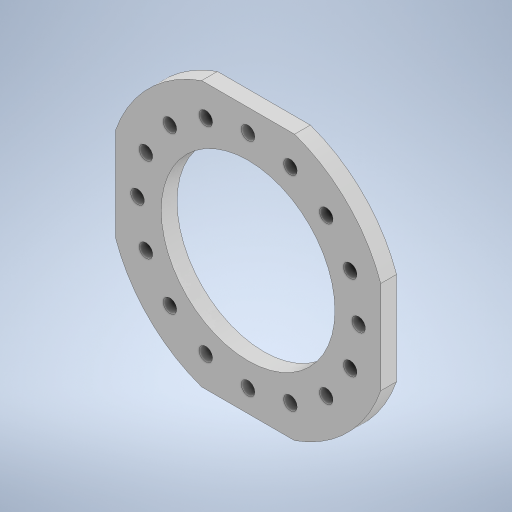
# Autodesk Inventor part: 감속기어1 - 하우징 커버
Saved by Autodesk Inventor 2023 (Build 270158000, 158)
## iProperties
Created: 2022-06-21
Part Number: 감속기어1 - 하우징 커버
Material: 일반
Document SubType Name: Modeling
Designer: user
Density: 1 g/cm^3
Appearance: 기본값
Author: user
Autodesk Inventor part; units mm, degrees
ref_plane "YZ Plane" through (0, 0, 0) normal (1, 0, 0) x (0, 1, 0)
ref_plane "XZ Plane" through (0, 0, 0) normal (0, 1, 0) x (-1, 0, 0)
ref_plane "XY Plane" through (0, 0, 0) normal (0, 0, 1) x (1, 0, 0)
sketch "스케치1" plane through (0, 0, 0) normal (0, 0, 1) x (1, 0, 0)
  circle A0 centre (0, 0) radius 44.5
  line L0 (-42, -42) -> (42, -42)
  line L1 (42, -42) -> (42, 42)
  line L2 (42, 42) -> (-42, 42)
  line L3 (-42, 42) -> (-42, -42)
  line L4 (-42, -42) -> (42, 42) construction
  line L5 (42, -42) -> (-42, 42) construction
  circle A1 centre (0, 0) radius 27.5
  point P0 (-42, 14.7054)
  point P1 (-42, -14.7054)
  point P2 (-14.7054, -42)
  point P3 (14.7054, -42)
  point P4 (42, -14.7054)
  point P5 (42, 14.7054)
  point P6 (14.7054, 42)
  point P7 (-14.7054, 42)
  dimension "d0" = 89
  dimension "d1" = 84
  dimension "d2" = 84
  dimension "d3" = 55
  constraints: 12 end point, 2 centre point, 2 coincident, 2 midpoint, 2 parallel, 1 horizontal, 1 perpendicular
  measures "d0" diameter of A0
  measures "d1" distance of L2.end L1.end
  measures "d2" distance of L1.end L0.end
  measures "d3" diameter of A1
extrude "돌출1" add sketch "스케치1" along normal blind 5 contours L1 A0 L0 L3 L2
sketch "스케치4" plane through (0, 0, 5) normal (0, 0, 1) x (1, 0, 0)
  circle A0 centre (0, 35) radius 2 construction
  circle A1 centre (0, 0) radius 33 construction
  circle A2 centre (0, 35) radius 2.15
  dimension "d25" = 4
  dimension "d26" = 66
  dimension "d27" = 4.3
  constraints: 3 centre point, 2 coincident, 1 tangent
  measures "d25" diameter of A0
  measures "d26" diameter of A1
  measures "d27" diameter of A2
extrude "돌출5" cut sketch "스케치4" against normal blind 10
pattern_circular "원형 패턴3" count 16 over 360 about axis through (0, 0, 0) along (0, 0, 1) of "돌출5"
